ring_v1 (Autodesk Fusion 360 design; units mm, degrees)
Autodesk Fusion 360 part; units mm, degrees
sketch "Skizze1" plane through (0, 0, 0) normal (0, 1, 0) x (1, 0, 0)
  ellipse E0 centre (13.5599, -15.1096) end of major axis (58.5014, -35.6433) minor radius 27.0113
  line L0 (-31.3816, 5.424) -> (58.5014, -35.6433) construction
  line L1 (2.3347, -39.678) -> (24.7851, 9.4587) construction
  ellipse E1 centre (13.5599, -15.1096) end of major axis (34.4101, -24.636) minor radius 19.9076
  line L2 (-7.2903, -5.5833) -> (34.4101, -24.636) construction
  line L3 (5.2869, -33.2167) -> (21.833, 2.9975) construction
  constraint coincident E0 L0.start
  constraint coincident E0 L0.end
  constraint coincident E0 L1.start
  constraint coincident E0 L1.end
  constraint concentric E0 E1
  constraint perpendicular L1 L2
  constraint coincident E1 L2.start
  constraint coincident E1 L2.end
  constraint coincident E1 L3.start
  constraint coincident E1 L3.end
cylinder "Grundkörper Zylinder1" add diameter 84.853 height 20 placed x (1, 0, 0) y (0, 0, -1) z (0, 1, 0) at (0, 0, 0) makes body 1
hole "Bohrung3" at (0, 20, 0) direction (0, -1, 0) diameter 40 depth 40 tip angle 118 bodies 1
thread "Gewinde1" "ISO Metric Trapezoidal Threads 28.0 TR28x3 7H" major diameter 28.5 minor diameter 25.1575 pitch 3 angle 60 modelled right hand crest width 0.375 on face at (1.9914, 6.6667, 19.9006) crest through (0, 21.6875, 12.5788) on bodies 1
cylinder "Grundkörper Zylinder2" add diameter 36.162 height 5 placed x (1, 0, 0) y (0, 0, -1) z (0, 1, 0) at (0, 0, 0) separate body makes body 2
hole "Bohrung4" at (0, 5, 0) direction (0, -1, 0) diameter 15 depth 15 tip angle 118 bodies 2
thread "Gewinde2" "ISO Metric Trapezoidal Threads 28.0 TR28x3 7H" major diameter 28.5 minor diameter 25.1575 pitch 3 angle 60 modelled right hand crest width 0.375 on face at (0.7468, 1.6667, 7.4627) crest through (0, 6.6875, 12.5788) on bodies 2
